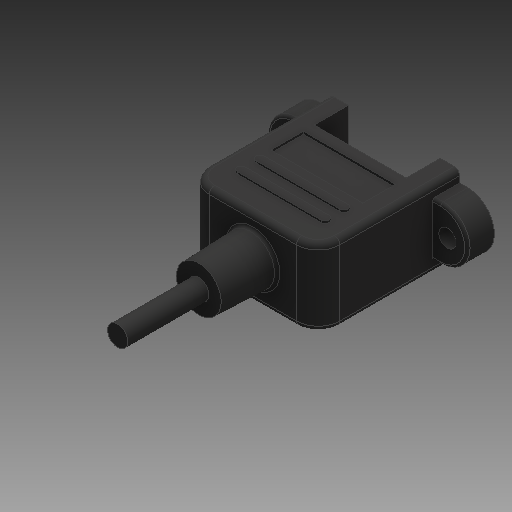
# Autodesk Inventor part: USB Cable B Male to B Female 90 degrees
Saved by Autodesk Inventor 2019 (Build 230136000, 136)
## iProperties
Created: 2017-10-16
Part Number: USB Cable B Male to B Female 90 degrees
Material: Nylon 6/6
Document SubType Name: Modeling
Designer: admin
Density: 1.13 g/cm^3
Appearance: Rubber - Black
Author: admin
Autodesk Inventor part; units mm, degrees
ref_plane "YZ Plane" through (0, 0, 0) normal (1, 0, 0) x (0, 1, 0)
ref_plane "XZ Plane" through (0, 0, 0) normal (0, 1, 0) x (-1, 0, 0)
sketch "Sketch1" plane through (0, 0, 0) normal (0, 0, 1) x (1, 0, 0)
  line L0 (8.075, -13.075) -> (-8.075, -13.075)
  line L1 (-12.075, -9.075) -> (-12.075, 13.075)
  line L2 (-12.075, 13.075) -> (12.075, 13.075)
  line L3 (12.075, 13.075) -> (12.075, -9.075)
  line L4 (12.075, -13.075) -> (-12.075, 13.075) construction
  line L5 (-12.075, -13.075) -> (12.075, 13.075) construction
  arc A0 (-12.075, -9.075) -> (-8.075, -13.075) centre (-8.075, -9.075) ccw
  arc A1 (8.075, -13.075) -> (12.075, -9.075) centre (8.075, -9.075) ccw
  point P0 (0, 0)
  dimension "d0" = 24.15
  dimension "d1" = 26.15
  dimension "d2" = 4
  constraints: 12 end point, 4 point on circle, 4 point on line, 4 tangent, 2 centre point, 2 midpoint, 2 parallel, 1 equal radius, 1 horizontal, 1 perpendicular
  measures "d0" distance of L1.end L2.end
  measures "d1" distance of L5.start L1.end
  measures "d2" radius of A0
extrude "Extrusion1" add sketch "Sketch1" along normal blind 14.2
sketch "Sketch2" plane through (-12.075, 13.075, 0) normal (0, 1, 0) x (1, 0, 0)
  line L0 (24.15, 0) -> (24.15, -14.2) construction
  line L1 (24.15, 0) -> (0, 0) construction
  line L2 (4, -14.2) -> (20.15, -14.2) construction
  line L3 (12.075, -14.2) -> (12.075, 8.7449) construction
  arc A0 (25.65, -12.05) -> (25.65, -2.15) centre (25.65, -7.1) ccw
  line L4 (24.15, 0) -> (24.15, -14.2) construction
  line L5 (24.15, -7.1) -> (-4.8998, -7.1) construction
  line L6 (30.6, -19.6482) -> (30.6, 9.5146) construction
  line L7 (25.65, -2.15) -> (24.15, -2.15)
  line L8 (25.65, -12.05) -> (24.15, -12.05)
  line L9 (24.15, -2.15) -> (24.15, -12.05)
  point P0 (12.075, 0)
  dimension "d5" = 9.9
  dimension "d6" = 6.45
  constraints: 12 end point, 3 horizontal, 3 point on line, 3 tangent, 2 midpoint, 2 point on circle, 2 vertical, 1 centre point, 1 collinear
  measures "d5" diameter of A0
  measures "d6" distance between parallel lines of L0 L6
extrude "Extrusion2" add sketch "Sketch2" against normal blind 5
sketch "Sketch3" plane through (-12.075, 8.075, 0) normal (0, -1, 0) x (1, 0, 0)
  line L0 (24.15, 8.6877) -> (26.9, 10.2754) construction
  line L1 (26.9, 10.2754) -> (29.65, 8.6877) construction
  line L2 (29.65, 8.6877) -> (29.65, 5.5123) construction
  line L3 (29.65, 5.5123) -> (26.9, 3.9246) construction
  line L4 (26.9, 3.9246) -> (24.15, 5.5123) construction
  line L5 (24.15, 5.5123) -> (24.15, 8.6877) construction
  line L6 (24.15, 2.15) -> (24.15, 12.05) construction
  arc A0 (25.65, 2.15) -> (25.65, 12.05) centre (25.65, 7.1) ccw construction
  line L7 (25.65, 7.1) -> (35.3892, 7.1) construction
  line L8 (26.9, 10.2754) -> (26.9, 3.9246) construction
  point P0 (12.075, 0)
  point P1 (26.9, 7.1)
  point P2 (26.9, 7.1)
  dimension "d9" = 5.5
  constraints: 16 end point, 2 point on line, 1 coincident, 1 collinear, 1 horizontal, 1 vertical, 13 other
  measures "d9" distance between parallel lines of L0 L3
sketch "Sketch4" plane through (-12.075, 8.075, 0) normal (0, -1, 0) x (1, 0, 0)
  circle A0 centre (26.9, 7.1) radius 1.6
  point P0 (12.075, 0)
  dimension "d10" = 3.2
  constraints: 1 centre point, 1 coincident
  measures "d10" diameter of A0
extrude "Extrusion3" cut sketch "Sketch4" against normal blind 5
mirror "Mirror1" about plane through (0, 0, 0) normal (1, 0, 0) of "Extrusion2", "Extrusion3"
sketch "Sketch5" plane through (-12.075, 13.075, 0) normal (0, 1, 0) x (1, 0, 0)
  line L0 (24.15, 0) -> (0, 0) construction
  line L1 (0, 0) -> (0, -2.15) construction
  line L2 (24.15, -14.2) -> (0, -14.2) projected
  line L3 (20.575, 0) -> (3.575, 0)
  line L4 (3.575, 0) -> (3.575, -14.2)
  line L5 (3.575, -14.2) -> (20.575, -14.2)
  line L6 (20.575, -14.2) -> (20.575, 0)
  line L7 (12.075, 0) -> (12.075, -22.6768) construction
  dimension "d13" = 17
  constraints: 10 end point, 2 parallel, 2 point on line, 1 horizontal, 1 perpendicular, 1 vertical, 1 other
  measures "d13" distance of L5.end L4.end
extrude "Extrusion4" cut sketch "Sketch5" against normal blind 6.3
sketch "Sketch6" plane through (-8.075, -13.075, 0) normal (0, -1, 0) x (1, 0, 0)
  circle A0 centre (8.075, 7.1) radius 4.5
  line L0 (0, 0) -> (16.15, 0) construction
  line L1 (20.15, 0) -> (20.15, 14.2) construction
  point P0 (8.075, 0)
  dimension "d16" = 9
  dimension "d17" = 7.1
  dimension "d18" = 12.075
  constraints: 1 centre point
  measures "d16" diameter of A0
  measures "d17" distance from line of L0 A0.centre
  measures "d18" distance from line of L1 A0.centre
extrude "Extrusion5" add sketch "Sketch6" along normal blind 10 draft -2
sketch "Sketch7" plane through (0, -23.075, 7.1) normal (0, -1, 0) x (1, 0, 0)
  circle A0 centre (0, 0) radius 4.1508 projected
  circle A1 centre (0, 0) radius 1.88
  point P0 (0, -7.1)
  dimension "d21" = 3.76
  constraints: 1 centre point, 1 coincident
  measures "d21" diameter of A1
extrude "Extrusion6" add sketch "Sketch7" along normal blind 15 contours A1
sketch "Sketch8" plane through (-12.075, 6.775, 0) normal (0, 1, 0) x (1, 0, 0)
  line L0 (3.575, -14.2) -> (3.575, 0) construction
  line L1 (3.575, 0) -> (20.575, 0) construction
  circle A0 centre (12.075, -7.1) radius 1.88 construction
  line L2 (18.135, -12.625) -> (6.015, -12.625)
  line L3 (6.015, -12.625) -> (6.015, -1.575)
  line L4 (6.015, -1.575) -> (18.135, -1.575)
  line L5 (18.135, -1.575) -> (18.135, -12.625)
  line L6 (18.135, -12.625) -> (6.015, -1.575) construction
  line L7 (6.015, -12.625) -> (18.135, -1.575) construction
  point P0 (12.075, 0)
  dimension "d24" = 12.12
  dimension "d25" = 11.05
  constraints: 12 end point, 2 midpoint, 2 parallel, 1 horizontal, 1 perpendicular
  measures "d24" distance of L3.end L4.end
  measures "d25" distance of L2.end L3.end
fillet "Fillet1" radius 1 10 edges at (-10.9034, -11.9034, 0) (0, -13.075, 0) (10.9034, -11.9034, 0) (12.075, 2, 0) (-12.075, 2, 0) (-10.9034, -11.9034, 14.2) (0, -13.075, 14.2) (10.9034, -11.9034, 14.2) (12.075, 2, 14.2) (-12.075, 2, 14.2)
sketch "Sketch9" plane through (0, 0, 0) normal (0, 0, -1) x (-1, 0, 0)
  line L0 (0, -48.305) -> (0, 23.305) construction
  line L1 (8.5, 4.775) -> (-8.5, 4.775)
  line L2 (-8.5, 4.775) -> (-8.5, -1.225)
  line L3 (-8.5, -1.225) -> (8.5, -1.225)
  line L4 (8.5, -1.225) -> (8.5, 4.775)
  line L5 (8.5, 4.775) -> (-8.5, -1.225) construction
  line L6 (-8.5, 4.775) -> (8.5, -1.225) construction
  line L7 (-8.5, 6.775) -> (8.5, 6.775) projected
  point P0 (0, 0)
  point P1 (0, 1.775)
  dimension "d27" = 17
  dimension "d28" = 6
  dimension "d29" = 2
  constraints: 12 end point, 2 midpoint, 2 parallel, 1 horizontal, 1 perpendicular, 1 point on line
  measures "d27" distance of L3.end L2.end
  measures "d28" distance of L2.end L1.end
  measures "d29" distance between parallel lines of L7 L1
extrude "Extrusion7" cut sketch "Sketch9" against normal blind 0.5
sketch "Sketch10" plane through (0, 0, 0) normal (0, 0, -1) x (-1, 0, 0)
  line L0 (8.5, -1.225) -> (-8.5, -1.225) construction
  line L1 (0, -48.305) -> (0, 23.305) construction
  line L2 (-7.75, -3.225) -> (7.75, -3.225)
  line L3 (8.5, -3.975) -> (8.5, -3.975)
  line L4 (7.75, -4.725) -> (-7.75, -4.725)
  line L5 (-8.5, -3.975) -> (-8.5, -3.975)
  line L6 (-8.5, -3.225) -> (8.5, -4.725) construction
  line L7 (8.5, -3.225) -> (-8.5, -4.725) construction
  line L8 (-7.75, -6.725) -> (7.75, -6.725)
  line L9 (8.5, -7.475) -> (8.5, -7.475)
  line L10 (7.75, -8.225) -> (-7.75, -8.225)
  line L11 (-8.5, -7.475) -> (-8.5, -7.475)
  line L12 (-8.5, -6.725) -> (8.5, -8.225) construction
  line L13 (8.5, -6.725) -> (-8.5, -8.225) construction
  arc A0 (7.75, -8.225) -> (8.5, -7.475) centre (7.75, -7.475) ccw
  arc A1 (8.5, -7.475) -> (7.75, -6.725) centre (7.75, -7.475) ccw
  arc A2 (-8.5, -7.475) -> (-7.75, -8.225) centre (-7.75, -7.475) ccw
  arc A3 (-7.75, -6.725) -> (-8.5, -7.475) centre (-7.75, -7.475) ccw
  arc A4 (-8.5, -3.975) -> (-7.75, -4.725) centre (-7.75, -3.975) ccw
  arc A5 (-7.75, -3.225) -> (-8.5, -3.975) centre (-7.75, -3.975) ccw
  arc A6 (8.5, -3.975) -> (7.75, -3.225) centre (7.75, -3.975) ccw
  arc A7 (7.75, -4.725) -> (8.5, -3.975) centre (7.75, -3.975) ccw
  point P0 (0, 0)
  point P1 (0, -3.975)
  point P2 (0, -7.475)
  dimension "d32" = 17
  dimension "d33" = 1.5
  dimension "d34" = 2
  dimension "d35" = 17
  dimension "d36" = 1.5
  dimension "d37" = 2
  dimension "d38" = 0.75
  constraints: 24 end point, 18 point on line, 16 point on circle, 16 tangent, 8 centre point, 7 equal radius, 4 midpoint, 4 parallel, 2 horizontal, 2 perpendicular
  measures "d32" distance of L6.end L7.end
  measures "d33" distance of L7.start L6.end
  measures "d34" distance between parallel lines of L0 L2
  measures "d35" distance of L12.end L13.end
  measures "d36" distance of L13.start L12.end
  measures "d37" distance between parallel lines of L4 L8
  measures "d38" radius of A0
extrude "Extrusion8" add sketch "Sketch10" along normal blind 0.4
ref_plane "Work Plane1" through (12.075, 8.075, 7.1) normal (0, 0, -1) x (-1, 0, 0)
mirror "Mirror2" about plane through (12.075, 8.075, 7.1) normal (0, 0, -1) of "Extrusion7", "Extrusion8"
fillet "Fillet2" radius 0.5 1 edges at (-4.5, -13.075, 7.1)
fillet "Fillet3" radius 0.5 6 edges at (-12.825, 8.075, 12.05) (-12.825, 8.075, 2.15) (-18.525, 8.075, 7.1) (12.825, 8.075, 12.05) (12.825, 8.075, 2.15) (18.525, 8.075, 7.1)
sketch "Sketch11" plane through (-12.075, 6.775, 0) normal (0, 1, 0) x (1, 0, 0)
  line L0 (7.575, -2.5467) -> (16.575, -2.5467)
  line L1 (16.575, -2.5467) -> (16.575, -11.5467)
  line L2 (16.575, -11.5467) -> (7.575, -11.5467)
  line L3 (7.575, -11.5467) -> (7.575, -2.5467)
  line L4 (7.575, -2.5467) -> (16.575, -11.5467) construction
  line L5 (16.575, -2.5467) -> (7.575, -11.5467) construction
  point P0 (12.075, 0)
  point P1 (12.075, -7.0467)
  dimension "d43" = 9
  dimension "d44" = 9
  constraints: 12 end point, 2 midpoint, 2 parallel, 1 horizontal, 1 perpendicular
  measures "d43" distance of L1.end L2.end
  measures "d44" distance of L0.end L1.end
extrude "Extrusion9" cut sketch "Sketch11" against normal blind 4
body "Solid1"
